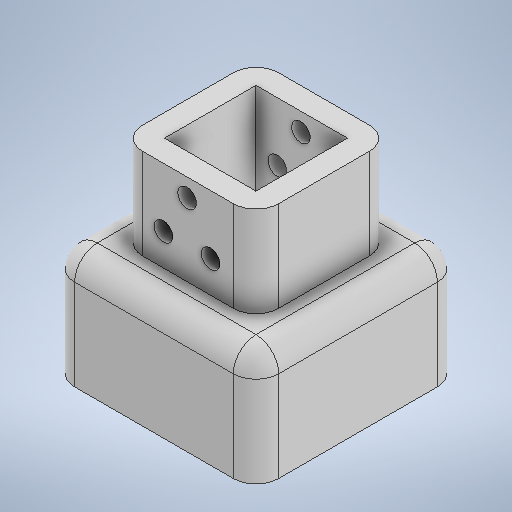
# Autodesk Inventor part: tool_shoe
Saved by Autodesk Inventor 2025 (Build 290162000, 162)
## iProperties
Created: 2025-01-20
Part Number: tool_shoe
Material: Generic
Document SubType Name: Modeling
Designer: danielrachi
Density: 1 g/cm^3
Appearance: Default
Author: danielrachi
Autodesk Inventor part; units mm, degrees
ref_plane "YZ Plane" through (0, 0, 0) normal (1, 0, 0) x (0, 1, 0)
ref_plane "XZ Plane" through (0, 0, 0) normal (0, 1, 0) x (-1, 0, 0)
ref_plane "XY Plane" through (0, 0, 0) normal (0, 0, 1) x (1, 0, 0)
sketch "Sketch2" plane through (0, 0, 0) normal (0, 1, 0) x (-1, 0, 0)
  line L0 (-10.1, 10.1) -> (10.1, 10.1)
  line L1 (10.1, 10.1) -> (10.1, -10.1)
  line L2 (10.1, -10.1) -> (-10.1, -10.1)
  line L3 (-10.1, -10.1) -> (-10.1, 10.1)
  line L4 (-10.1, 10.1) -> (10.1, -10.1) construction
  line L5 (10.1, 10.1) -> (-10.1, -10.1) construction
  line L6 (-15, 15) -> (15, 15)
  line L7 (15, 15) -> (15, -15)
  line L8 (15, -15) -> (-15, -15)
  line L9 (-15, -15) -> (-15, 15)
  line L10 (-15, 15) -> (15, -15) construction
  line L11 (15, 15) -> (-15, -15) construction
  point P0 (0, 0)
  dimension "d2" = 20.2
  dimension "d3" = 20.2
  dimension "d4" = 30
  dimension "d5" = 30
  constraints: 24 end point, 4 midpoint, 4 parallel, 2 horizontal, 2 perpendicular
  measures "d2" distance of L1.end L2.end
  measures "d3" distance of L0.end L1.end
  measures "d4" distance of L7.end L8.end
  measures "d5" distance of L6.end L7.end
extrude "Extrusion1" add sketch "Sketch2" along normal blind 20
sketch "Sketch3" plane through (-10.1, 0, -10.1) normal (0, 0, 1) x (1, 0, 0)
  circle A0 centre (9.9, 16) radius 2.05
  circle A1 centre (4.7038, 7) radius 2.05
  circle A2 centre (15.0962, 7) radius 2.05
  point P0 (10.1, 0)
  point P1 (9.9, 10)
  dimension "d8" = 4.1
  dimension "d9" = 6
  dimension "d12" = 360
  constraints: 3 centre point, 7 other
  measures "d8" diameter of A0
  measures "d9" distance of point (9.9, 10) A0.centre
extrude "Extrusion2" cut sketch "Sketch3" along normal through all both and the other way through all
sketch "Sketch4" plane through (0, 0, 0) normal (0, -1, 0) x (1, 0, 0)
  line L0 (-22.5, -22.5) -> (22.5, -22.5)
  line L1 (22.5, -22.5) -> (22.5, 22.5)
  line L2 (22.5, 22.5) -> (-22.5, 22.5)
  line L3 (-22.5, 22.5) -> (-22.5, -22.5)
  line L4 (-22.5, -22.5) -> (22.5, 22.5) construction
  line L5 (22.5, -22.5) -> (-22.5, 22.5) construction
  point P0 (0, 0)
  dimension "d16" = 45
  dimension "d17" = 45
  constraints: 12 end point, 2 midpoint, 2 parallel, 1 horizontal, 1 perpendicular
  measures "d16" distance of L2.end L1.end
  measures "d17" distance of L1.end L0.end
extrude "Extrusion3" add sketch "Sketch4" along normal blind 25
sketch "Sketch5" plane through (0, -25, 0) normal (0, -1, 0) x (1, 0, 0)
  circle A0 centre (0, 0) radius 20
  line L0 (-20, 0) -> (20, 0)
  dimension "d20" = 40
  constraints: 2 end point, 2 point on circle, 1 centre point, 1 coincident, 1 horizontal
  measures "d20" diameter of A0
revolve "Revolution1" cut sketch "Sketch5" angle 360 about axis through (-20, -25, 0) along (1, 0, 0) picked at (4.9901, 4.4208) contours L0 A0
fillet "Fillet1" radius 5 12 edges at (22.5, -12.5, 22.5) (-22.5, -12.5, 22.5) (22.5, -12.5, -22.5) (-22.5, -12.5, -22.5) (0, 0, 22.5) (22.5, 0, 0) (0, 0, -22.5) (-22.5, 0, 0) (15, 10, 15) (15, 10, -15) (-15, 10, 15) (-15, 10, -15)
equation "\"d2\" = tool_mount_side + clearance"
equation "\"d3\" = tool_mount_side + clearance"
equation "\"d6\" = tool_mount_depth"
equation "\"tool_mount_side\" = 20"
equation "\"clearance\" = 0.2"
equation "\"tool_mount_depth\" = 20"
body "Solid1"
